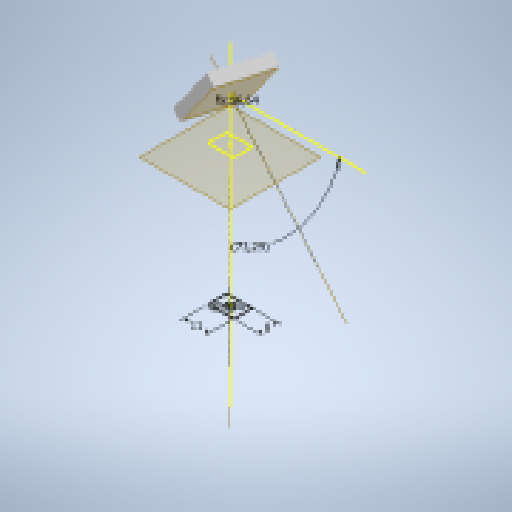
# Autodesk Inventor part: wyliczenia
Saved by Autodesk Inventor 2025.1 (Build 291241000, 241)
## iProperties
Created: 2024-10-30
Part Number: wyliczenia
Material: Ogólny
Document SubType Name: Modeling
Designer: PC
Density: 1 g/cm^3
Appearance: Domyślna
Author: PC
Autodesk Inventor part; units mm, degrees
ref_plane "YZ Plane" through (0, 0, 0) normal (1, 0, 0) x (0, 1, 0)
sketch "Szkic1" plane through (0, 0, 0) normal (0, 1, 0) x (-1, 0, 0)
  line L0 (5.5, -4) -> (-5.5, -4)
  line L1 (-5.5, -4) -> (-5.5, 4)
  line L2 (-5.5, 4) -> (5.5, 4)
  line L3 (5.5, 4) -> (5.5, -4)
  line L4 (5.5, -4) -> (-5.5, 4) construction
  line L5 (13.1739, -13.1739) -> (-22.2043, 22.2043) construction
  point P0 (0, 0)
  dimension "d0" = 11
  dimension "d1" = 8
  dimension "d2" = 45
  constraints: 12 end point, 2 parallel, 1 horizontal, 1 midpoint, 1 perpendicular, 1 point on line
  measures "d0" distance of L1.end L2.end
  measures "d1" distance of L0.end L1.end
  measures "d2" angle of L2 L5
ref_plane "Płaszczyzna konstrukcyjna1" through (-13.1739, 0, -13.1739) normal (-0.7071, 0, 0.7071) x (0.7071, 0, 0.7071)
sketch "Szkic2" plane through (-13.1739, 0, -13.1739) normal (-0.7071, 0, 0.7071) x (0.7071, 0, 0.7071)
  line L0 (18.6307, 0) -> (10.6505, 17.9239) construction
  line L1 (18.6307, -12) -> (18.6307, 72) construction
  dimension "d3" = 24
  constraints: 2 end point
  measures "d3" angle of L1 L0
ref_plane "Płaszczyzna konstrukcyjna2" through (0, 60, 0) normal (0, 1, 0) x (-1, 0, 0)
sketch "Szkic3" plane through (0, 60, 0) normal (0, 1, 0) x (-1, 0, 0)
  line L0 (-34.8726, 34.8726) -> (27.8498, -27.8498) construction
  point P0 (0, 0)
ref_plane "Płaszczyzna konstrukcyjna3" through (-18.8895, 60, -18.8895) normal (0, 0.3003, 0.9538) x (1, 0, 0)
sketch "Szkic5" plane through (-18.8895, 60, -18.8895) normal (0, 0.3003, 0.9538) x (1, 0, 0)
  line L0 (-9.7019, 0) -> (58.2115, 0) projected
  line L1 (27.8115, -92.6142) -> (-4.6352, 15.4357) projected
  line L2 (0, 0) -> (48.5096, -36.0825) construction
  point P0 (18.8895, -62.9032)
  dimension "d5" = 36.643
  dimension "d6" = 73.285
  constraints: 2 end point, 2 point on line
  measures "d5" angle of L0 L2
  measures "d6" angle of L1 L0
sketch "Szkic6" plane through (0, 60, 0) normal (0, 1, 0) x (-1, 0, 0)
  line L0 (-5.5, 4) -> (5.5, 4) projected
  line L1 (-5.5, -4) -> (-5.5, 4) projected
  line L2 (5.5, 4) -> (5.5, -4) projected
  line L3 (5.5, -4) -> (-5.5, -4) projected
  point P0 (0, 0)
ref_plane "Płaszczyzna konstrukcyjna4" through (-18.8895, 60, -18.8895) normal (0.8024, -0.5693, 0.1792) x (0.5786, 0.8156, 0)
sketch "Szkic7" plane through (-18.8895, 60, -18.8895) normal (0.8024, -0.5693, 0.1792) x (0.5786, 0.8156, 0)
  line L0 (11.5, -11.5) -> (-11.5, -11.5)
  line L1 (-11.5, -11.5) -> (-11.5, 11.5)
  line L2 (-11.5, 11.5) -> (11.5, 11.5)
  line L3 (11.5, 11.5) -> (11.5, -11.5)
  point P0 (-38.0044, 9.6002)
  point P1 (0, 0)
  point P2 (0, -11.5)
  point P3 (-11.5, 0)
  dimension "d7" = 23
  dimension "d8" = 23
  constraints: 8 end point, 2 midpoint, 2 parallel, 1 horizontal, 1 horizontal alignment, 1 perpendicular, 1 vertical alignment
  measures "d7" distance of L1.end L2.end
  measures "d8" distance of L0.end L1.end
extrude "Wyciągnięcie proste1" add sketch "Szkic7" against normal blind 1.2
equation "\"d5\" = 0.5 * d6"
